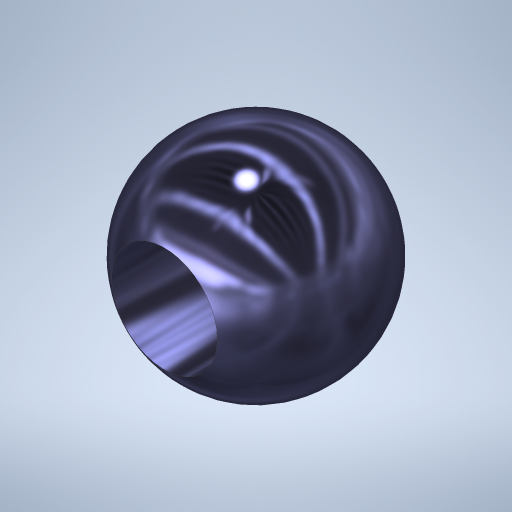
# Autodesk Inventor part: 0.25 Ball
Saved by Autodesk Inventor 2023.1 (Build 271208000, 208)
## iProperties
Created: 2019-11-29
Part Number: 0.25 Ball
Material: Generic
Document SubType Name: Modeling
Designer: Jopa
Density: 1 g/cm^3
Appearance: Default
Author: Jopa
Autodesk Inventor part; units mm, degrees
ref_plane "YZ Plane" through (0, 0, 0) normal (1, 0, 0) x (0, 1, 0)
ref_plane "XZ Plane" through (0, 0, 0) normal (0, 1, 0) x (-1, 0, 0)
ref_plane "XY Plane" through (0, 0, 0) normal (0, 0, 1) x (1, 0, 0)
sketch "Sketch1" plane through (0, 0, 0) normal (0, 0, 1) x (1, 0, 0)
  line L0 (-4.1275, 0) -> (2.54, 0) construction
  line L1 (0, -4.445) -> (0, 4.445) projected
  circle A0 centre (0, 0) radius 1.5875
  arc A1 (0, 3.175) -> (0, -3.175) centre (0, 0) ccw
  line L2 (0, 3.175) -> (0, -3.175)
  dimension "d0" = 3.175
  dimension "d1" = 6.35
  constraints: 2 centre point, 2 coincident, 2 end point, 2 point on circle, 2 point on line, 1 vertical
  measures "d0" diameter of A0
  measures "d1" diameter of A1
revolve "Revolution1" add sketch "Sketch1" angle 360 about axis through (0, -10, 0) along (0, 1, 0) picked at (-0.4948, -0.1876) contours A1 L1 A0 | A0 L1
extrude "Extrusion1" cut sketch "Sketch1" along normal through all both and the other way through all contours A0 L1 | L1 A0
body "Solid1"
